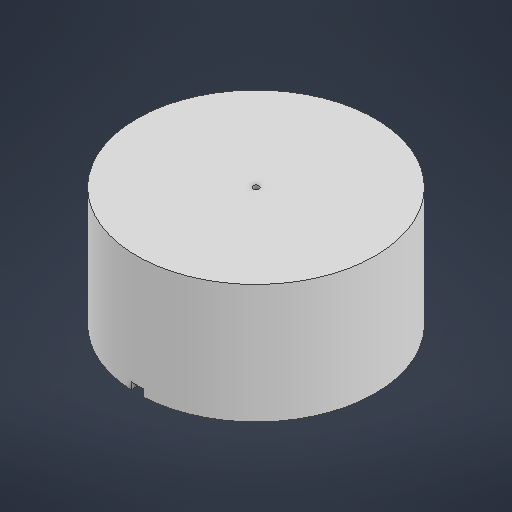
# Autodesk Inventor part: Base
Saved by Autodesk Inventor 2027.1 (Build 311267000, 267)
## iProperties
Created: 2026-10-01
Part Number: Base
Material: Generic
Document SubType Name: Modeling
Designer: HP
Density: 1 g/cm^3
Appearance: Default
Author: HP
Autodesk Inventor part; units mm, degrees
ref_plane "YZ Plane" through (0, 0, 0) normal (1, 0, 0) x (0, 1, 0)
ref_plane "XZ Plane" through (0, 0, 0) normal (0, 1, 0) x (-1, 0, 0)
ref_plane "XY Plane" through (0, 0, 0) normal (0, 0, 1) x (1, 0, 0)
sketch "Sketch1" plane through (0, 0, 0) normal (0, 1, 0) x (-1, 0, 0)
  circle A0 centre (0, 0) radius 100
  dimension "d0" = 200
  constraints: 1 centre point, 1 coincident
  measures "d0" diameter of A0
extrude "Extrusion1" add sketch "Sketch1" along normal blind 100
sketch "Sketch2" plane through (0, 100, 0) normal (0, 1, 0) x (1, 0, 0)
  circle A0 centre (0, 0) radius 2.5
  dimension "d3" = 5
  constraints: 1 centre point, 1 coincident
  measures "d3" diameter of A0
extrude "Extrusion2" cut sketch "Sketch2" along normal blind 22
sketch "Sketch6" plane through (0, 0, 0) normal (0, -1, 0) x (1, 0, 0)
  line L0 (15.5, 15.5) -> (-15.5, 15.5)
  line L1 (-15.5, 15.5) -> (-15.5, -15.5)
  line L2 (-15.5, -15.5) -> (15.5, -15.5)
  line L3 (15.5, -15.5) -> (15.5, 15.5)
  line L4 (15.5, 15.5) -> (-15.5, -15.5) construction
  line L5 (-15.5, 15.5) -> (15.5, -15.5) construction
  line L6 (21.15, 21.15) -> (-21.15, 21.15)
  line L7 (-21.15, 21.15) -> (-21.15, -21.15)
  line L8 (-21.15, -21.15) -> (21.15, -21.15)
  line L9 (21.15, -21.15) -> (21.15, 21.15)
  line L10 (21.15, 21.15) -> (-21.15, -21.15) construction
  line L11 (-21.15, 21.15) -> (21.15, -21.15) construction
  circle A0 centre (-15.5, -15.5) radius 1.4
  circle A1 centre (-15.5, 15.5) radius 1.4
  circle A2 centre (15.5, 15.5) radius 1.4
  circle A3 centre (15.5, -15.5) radius 1.4
  point P0 (0, 0)
  dimension "d18" = 31
  dimension "d19" = 31
  dimension "d21" = 42.3
  dimension "d22" = 42.3
  dimension "d23" = 2.8
  dimension "d24" = 2.8
  dimension "d25" = 2.8
  dimension "d26" = 2.8
  constraints: 24 end point, 4 centre point, 4 midpoint, 4 parallel, 2 horizontal, 2 perpendicular, 1 coincident
  measures "d18" distance of L2.end L1.end
  measures "d19" distance between parallel lines of L2 L0
  measures "d21" distance of L8.end L7.end
  measures "d22" distance of L7.end L6.end
  measures "d23" diameter of A0
  measures "d24" diameter of A1
  measures "d25" diameter of A2
  measures "d26" diameter of A3
extrude "Extrusion5" cut sketch "Sketch6" against normal blind 22 contours L0 A2 L3 A3 L2 A0 L1 A1 | L9 L8 L7 L6
sketch "Sketch7" plane through (0, 22, 0) normal (0, -1, 0) x (1, 0, 0)
  circle A0 centre (0, 0) radius 2.5 projected
  circle A1 centre (0, 0) radius 2.5
  dimension "d29" = 5
  constraints: 1 centre point, 1 coincident
  measures "d29" diameter of A1
extrude "Extrusion6" cut sketch "Sketch7" against normal blind 80
sketch "Sketch8" plane through (0, 22, 0) normal (0, -1, 0) x (1, 0, 0)
  circle A0 centre (0, 0) radius 11
  dimension "d32" = 22
  constraints: 1 centre point, 1 coincident
  measures "d32" diameter of A0
extrude "Extrusion7" cut sketch "Sketch8" against normal blind 2
sketch "Sketch9" plane through (0, 0, 0) normal (0, -1, 0) x (1, 0, 0)
  line L0 (-21.15, 21.15) -> (21.15, 21.15) projected
  circle A0 centre (0, 0) radius 100 projected
  line L1 (5.3123, 21.15) -> (-5.021, 21.15)
  line L2 (-5.021, 99.8739) -> (5.3123, 99.8739)
  line L3 (-5.021, 21.15) -> (-0.021, 21.15)
  line L4 (-0.021, 99.8739) -> (-5.021, 99.8739)
  line L5 (5.3123, 21.15) -> (-5.021, 21.15)
  line L6 (-5.021, 21.15) -> (-5.021, 99.8739)
  line L7 (-5.021, 99.8739) -> (5.3123, 99.8739)
  line L8 (5.3123, 99.8739) -> (5.3123, 21.15)
  arc A1 (5.3123, 99.8739) -> (-5.021, 99.8739) centre (0.1457, 63.1234) ccw
  point P0 (5.021, 99.8739)
  point P1 (5.3123, 99.8588)
  dimension "d40" = 78.7239
  constraints: 16 end point, 4 parallel, 3 horizontal, 2 point on circle, 2 point on line, 1 centre point, 1 perpendicular, 2 other
  measures "d40" distance of L5.end L4.end
extrude "Extrusion8" cut sketch "Sketch9" against normal blind 6 contours L6 L2 A0 L8 L0 | A1 L2 A0 | A0 L2
equation "\"d24\" = d23"
equation "\"d25\" = d23"
equation "\"d26\" = d23"
body "Solid1"
